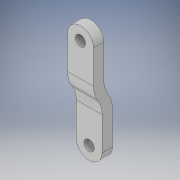
# Autodesk Inventor part: jumelo
Saved by Autodesk Inventor 2017 (Build 210142000, 142)
## iProperties
Created: 2019-10-14
Part Number: jumelo
Material: Generic
Document SubType Name: Modeling
Designer: 20171enpro0154
Density: 1 g/cm^3
Appearance: Default
Author: 20171enpro0154
Autodesk Inventor part; units mm, degrees
ref_plane "YZ Plane" through (0, 0, 0) normal (1, 0, 0) x (0, 1, 0)
ref_plane "XZ Plane" through (0, 0, 0) normal (0, 1, 0) x (-1, 0, 0)
ref_plane "XY Plane" through (0, 0, 0) normal (0, 0, 1) x (1, 0, 0)
sketch "Sketch1" plane through (0, 0, 0) normal (1, 0, 0) x (0, 1, 0)
  line L0 (0, 4.3301) -> (0, 35)
  line L1 (0, 35) -> (6, 35)
  line L2 (6, 35) -> (6, 4.3301)
  line L3 (5, -4.3301) -> (5, -35)
  line L4 (5, -35) -> (11, -35)
  line L5 (11, -35) -> (11, -4.3301)
  line L6 (0, 4.3301) -> (5, -4.3301)
  line L7 (2.5, 0) -> (6, 0) construction
  line L8 (6, 4.3301) -> (11, -4.3301)
  point P0 (0, 0)
  dimension "d1" = 6
  dimension "d11" = 6
  constraints: 18 end point, 3 perpendicular, 2 vertical, 1 coincident, 1 horizontal, 1 midpoint
  measures "d1" distance of L0.end L1.end
  measures "d11" distance of L3.end L4.end
extrude "Extrusão1" add sketch "Sketch1" along normal blind 15
fillet "Arredondamento1" radius 15 4 edges at (7.5, 11, -4.3301) (7.5, 6, 4.3301) (7.5, 0, 4.3301) (7.5, 5, -4.3301)
fillet "Arredondamento2" radius 7.5 4 edges at (15, 3, 35) (0, 3, 35) (15, 8, -35) (0, 8, -35)
sketch "Esboço2" plane through (0, 0, 8.3494) normal (0, -1, 0) x (1, 0, 0)
  line L0 (0, -9.1987) -> (15, -9.1987) projected
  arc A0 (15, 19.1506) -> (0, 19.1506) centre (7.5, 19.1506) ccw projected
  arc A1 (0, -35.8494) -> (15, -35.8494) centre (7.5, -35.8494) ccw projected
  circle A2 centre (7.5, 19.1506) radius 3
  circle A3 centre (7.5, -35.8494) radius 3
  point P0 (0, -8.3494)
  dimension "d29" = 6
  dimension "d31" = 6
  constraints: 2 centre point, 2 coincident
  measures "d29" diameter of A2
  measures "d31" diameter of A3
hole "Furo1" at (7.5, 0, 27.5) at (7.5, 0, -27.5) direction (0, 1, 0) diameter 6 end through all
